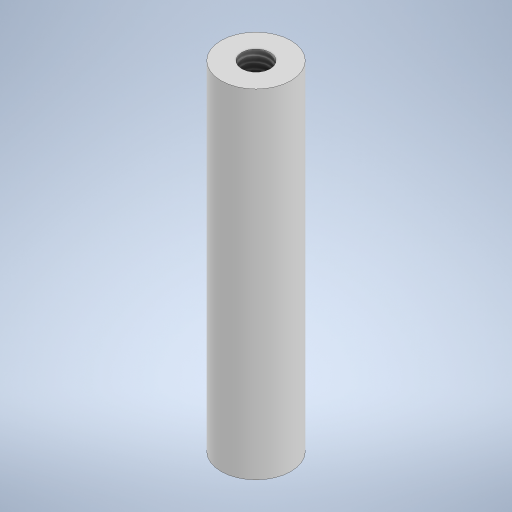
# Autodesk Inventor part: Connecting Rod
Saved by Autodesk Inventor 2023 (Build 270158000, 158)
## iProperties
Created: 2023-01-05
Part Number: Connecting Rod
Material: Generic
Document SubType Name: Modeling
Designer: Hayden Swanson
Density: 1 g/cm^3
Appearance: Default
Author: Hayden Swanson
Autodesk Inventor part; units mm, degrees
ref_plane "YZ Plane" through (0, 0, 0) normal (1, 0, 0) x (0, 1, 0)
ref_plane "XZ Plane" through (0, 0, 0) normal (0, 1, 0) x (-1, 0, 0)
ref_plane "XY Plane" through (0, 0, 0) normal (0, 0, 1) x (1, 0, 0)
sketch "Sketch1" plane through (0, 0, 0) normal (0, 1, 0) x (-1, 0, 0)
  circle A0 centre (0, 0) radius 3.0734
  dimension "d0" = 6.1468
  constraints: 1 centre point, 1 coincident
  measures "d0" diameter of A0
extrude "Extrusion1" add sketch "Sketch1" along normal blind 29.845
sketch "Sketch2" plane through (0, 29.845, 0) normal (0, 1, 0) x (1, 0, 0)
  circle A0 centre (0, 0) radius 1.2573
  dimension "d6" = 2.5146
  constraints: 1 centre point, 1 coincident
  measures "d6" diameter of A0
extrude "Extrusion2" cut sketch "Sketch2" against normal blind 9.652
thread "Thread2" size "3-48 UNC" class "2B" standard "ANSI Unified Screw Threads" length 88.9
sketch "Sketch3" plane through (0, 0, 0) normal (0, -1, 0) x (1, 0, 0)
  circle A0 centre (0, 0) radius 1.2573
  dimension "d11" = 2.5146
  constraints: 1 centre point, 1 coincident
  measures "d11" diameter of A0
extrude "Extrusion3" cut sketch "Sketch3" against normal blind 9.652
thread "Thread3" size "3-48 UNC" class "2B" standard "ANSI Unified Screw Threads" length 88.9
body "Solid1"
